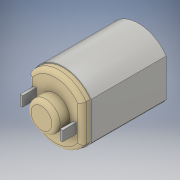
# Autodesk Inventor part: J024 motor
Saved by Autodesk Inventor 2016 SP1 (Build 200210100, 210)
## iProperties
Created: 2016-09-17
Part Number: J024 motor
Material: Generic
Document SubType Name: Modeling
Designer: benja
Density: 1 g/cm^3
Appearance: Default
Author: benja
Autodesk Inventor part; units mm, degrees
ref_plane "YZ Plane" through (0, 0, 0) normal (1, 0, 0) x (0, 1, 0)
ref_plane "XZ Plane" through (0, 0, 0) normal (0, 1, 0) x (-1, 0, 0)
ref_plane "XY Plane" through (0, 0, 0) normal (0, 0, 1) x (1, 0, 0)
sketch "Sketch1" plane through (0, 0, 0) normal (0, 0, 1) x (1, 0, 0)
  point P0 (0, 0)
sketch "Sketch2" plane through (0, 0, 0) normal (0, 0, 1) x (1, 0, 0)
  line L0 (-3.3, 2.2605) -> (-3.3, -2.2605)
  line L1 (3.3, 2.2605) -> (3.3, -2.2605)
  arc A0 (-3.3, -2.2605) -> (3.3, -2.2605) centre (0, 0) ccw
  arc A1 (3.3, 2.2605) -> (-3.3, 2.2605) centre (0, 0) ccw
  dimension "d1" = 6.6
  dimension "d2" = 4
  constraints: 4 end point, 4 point on circle, 2 centre point, 2 parallel, 1 coincident, 1 concentric, 1 vertical
  measures "d1" distance between parallel lines of L1 L0
  measures "d2" radius of A1
extrude "Extrusion1" add sketch "Sketch2" along normal blind 9
sketch "Sketch3" plane through (0, 0, 9) normal (0, 0, 1) x (1, 0, 0)
  point P0 (0, 0)
sketch "Sketch4" plane through (0, 0, 9) normal (0, 0, 1) x (1, 0, 0)
  line L0 (-3.3, 2.2605) -> (-3.3, -2.2605) projected
  arc A0 (-3.3, -2.2605) -> (3.3, -2.2605) centre (0, 0) ccw projected
  line L1 (3.3, -2.2605) -> (3.3, 2.2605) projected
  arc A1 (3.3, 2.2605) -> (-3.3, 2.2605) centre (0, 0) ccw projected
  line L2 (-3.2, 2.2293) -> (-3.2, -2.2293)
  arc A2 (-3.2, -2.2293) -> (3.2, -2.2293) centre (0, 0) ccw
  line L3 (3.2, -2.2293) -> (3.2, 2.2293)
  arc A3 (3.2, 2.2293) -> (-3.2, 2.2293) centre (0, 0) ccw
  dimension "d5" = 0.1
  constraints: 4 end point, 4 point on circle, 2 centre point, 3 other
  measures "d5" radial gap between concentric circles of A1 A3
extrude "Extrusion2" add sketch "Sketch4" along normal blind 1 contours A3 L3 A2 L2
fillet "Fillet1" radius 0.5 4 edges at (3.2, 0, 10) (0, 3.9, 10) (-3.2, 0, 10) (0, -3.9, 10)
sketch "Sketch5" plane through (0, 0, 10) normal (0, 0, 1) x (1, 0, 0)
  circle A0 centre (0, 0) radius 1.75
  dimension "d9" = 3.5
  constraints: 1 centre point, 1 coincident
  measures "d9" diameter of A0
extrude "Extrusion3" add sketch "Sketch5" along normal blind 1.65
fillet "Fillet2" radius 0.5 1 edges at (-1.75, 0, 11.65)
sketch "Sketch6" plane through (0, 0, 10) normal (0, 0, 1) x (1, 0, 0)
  line L0 (2.25, -1.2) -> (2.55, -1.2)
  line L1 (2.55, -1.2) -> (2.55, 0)
  line L2 (2.55, 0) -> (2.25, 0)
  line L3 (2.25, 0) -> (2.25, -1.2)
  circle A0 centre (0, 0) radius 1.75 projected
  line L4 (-2.55, 0) -> (-2.25, 0)
  line L5 (-2.25, 0) -> (-2.25, 1.2)
  line L6 (-2.25, 1.2) -> (-2.55, 1.2)
  line L7 (-2.55, 1.2) -> (-2.55, 0)
  point P0 (1.4682, 1.2)
  dimension "d13" = 0.3
  dimension "d14" = 1.2
  dimension "d15" = 0.5
  dimension "d16" = 0.3
  dimension "d17" = 1.2
  dimension "d18" = 0.5
  constraints: 16 end point, 4 parallel, 3 point on line, 2 horizontal, 2 perpendicular
  measures "d13" distance of L2.end L1.end
  measures "d14" distance of L1.end L0.end
  measures "d15" distance edge to line of A0 L3
  measures "d16" distance of L6.end L5.end
  measures "d17" distance of L5.end L4.end
  measures "d18" distance edge to line of A0 L5
extrude "Extrusion4" add sketch "Sketch6" along normal blind 1.65 contours L3 L2 L1 L0 | L7 L6 L5 L4
body "Solid1"
